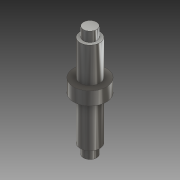
# Autodesk Inventor part: shaft_1_2
Saved by Autodesk Inventor 2017 SP1 (Build 210196100, 196)
## iProperties
Created: 2017-06-05
Part Number: shaft_1_2
Material: Generic
Document SubType Name: Modeling
Designer: Tomasz
Density: 1 g/cm^3
Appearance: Steel - Polished
Author: Tomasz
Autodesk Inventor part; units mm, degrees
ref_plane "YZ Plane" through (0, 0, 0) normal (1, 0, 0) x (0, 1, 0)
ref_plane "XZ Plane" through (0, 0, 0) normal (0, 1, 0) x (-1, 0, 0)
ref_plane "XY Plane" through (0, 0, 0) normal (0, 0, 1) x (1, 0, 0)
sketch "Sketch1" plane through (0, 0, 0) normal (0, 1, 0) x (-1, 0, 0)
  line L0 (0, 0) -> (1, 0)
  line L1 (1, 0) -> (1, -1.5)
  line L2 (1, -1.5) -> (1.5, -1.5)
  line L3 (1.5, -6.85) -> (2.5, -6.85)
  line L4 (2.5, -6.85) -> (2.5, -8.85)
  line L5 (2.5, -8.85) -> (1.5, -8.85)
  line L6 (1.5, -8.85) -> (1.5, -15.2007)
  line L7 (1, -17) -> (0, -17)
  line L8 (0, 0) -> (0, -17)
  line L9 (1.4788, -15.5) -> (1, -15.5)
  line L10 (1, -15.5) -> (1, -17)
  line L11 (1.4788, -15.5) -> (1.5, -15.5)
  line L12 (1.5, -1.5) -> (1.5, -6.85)
  line L13 (1.5, -6.85) -> (1.5, -1.5)
  line L14 (1.5, -15.5) -> (1.5, -15.2007)
  line L15 (1.5, -15.2007) -> (1.5, -15.2007)
  dimension "d1" = 1.5
  dimension "d4" = 2
  dimension "d19" = 14
  dimension "d21" = 1.5
  dimension "d30" = 2
  dimension "d31" = 2
  dimension "d33" = 3
  dimension "d34" = 5
  dimension "d35" = 3
  dimension "d37" = 0.2993
  dimension "d38" = 3
  dimension "d42" = 5.35
  constraints: 32 end point, 6 perpendicular, 3 horizontal, 3 point on line, 2 vertical
  measures "d1" distance between parallel lines of L2 L0
  measures "d4" distance between parallel lines of L5 L3
  measures "d19" distance between parallel lines of L9 L2
  measures "d21" distance between parallel lines of L9 L7
  measures "d30" diameter of L1 L8
  measures "d31" diameter of L10 L8
  measures "d33" diameter of L6 L8
  measures "d34" diameter of L4 L8
  measures "d35" diameter of L12 L8
  measures "d37" distance between parallel lines of L11 L15
  measures "d38" diameter of L14 L8
  measures "d42" distance between parallel lines of L3 L2
revolve "Revolution1" add sketch "Sketch1" angle 360 about axis through (0, 0, 0) along (0, 0, -1)
body "Solid1"
